Autodesk Fusion 360 part; units mm, degrees
(part 3 of 7)
  line L360 (75.0921, -60.7097) -> (75.2145, -60.5939)
  line L361 (75.2145, -60.5939) -> (75.3304, -60.4715)
  line L362 (75.3304, -60.4715) -> (75.4394, -60.343)
  line L363 (75.4394, -60.343) -> (75.6678, -60.5263)
  line L364 (75.6678, -60.5263) -> (75.7289, -60.5629)
  line L365 (75.7289, -60.5629) -> (75.7952, -60.5929)
  line L366 (75.7952, -60.5929) -> (75.865, -60.6184)
  line L367 (75.865, -60.6184) -> (75.9376, -60.6398)
  line L368 (75.9376, -60.6398) -> (76.0128, -60.6576)
  line L369 (76.0128, -60.6576) -> (76.0901, -60.672)
  line L370 (76.0901, -60.672) -> (76.1695, -60.6831)
  line L371 (76.1695, -60.6831) -> (76.2508, -60.6908)
  line L372 (76.2508, -60.6908) -> (76.3338, -60.6954)
  line L373 (76.3338, -60.6954) -> (76.4183, -60.6968)
  line L374 (76.4183, -60.6968) -> (76.5044, -60.695)
  line L375 (76.5044, -60.695) -> (76.5918, -60.69)
  line L376 (76.5918, -60.69) -> (76.66, -60.5798)
  line L377 (76.66, -60.5798) -> (76.7248, -60.4675)
  line L378 (76.7248, -60.4675) -> (76.7861, -60.3533)
  line L379 (76.7861, -60.3533) -> (76.7467, -60.2752)
  line L380 (76.7467, -60.2752) -> (76.7053, -60.1998)
  line L381 (76.7053, -60.1998) -> (76.6618, -60.1272)
  line L382 (76.6618, -60.1272) -> (76.6164, -60.0576)
  line L383 (76.6164, -60.0576) -> (76.569, -59.9911)
  line L384 (76.569, -59.9911) -> (76.5197, -59.9279)
  line L385 (76.5197, -59.9279) -> (76.4686, -59.8681)
  line L386 (76.4686, -59.8681) -> (76.4156, -59.8119)
  line L387 (76.4156, -59.8119) -> (76.3607, -59.7598)
  line L388 (76.3607, -59.7598) -> (76.3038, -59.7121)
  line L389 (76.3038, -59.7121) -> (76.2446, -59.6697)
  line L390 (76.2446, -59.6697) -> (76.1824, -59.635)
  line L391 (76.1824, -59.635) -> (75.9094, -59.5289)
  line L392 (75.9094, -59.5289) -> (75.9662, -59.3702)
  line L393 (75.9662, -59.3702) -> (76.0142, -59.2086)
  line L394 (76.0142, -59.2086) -> (76.0534, -59.0447)
  line L395 (76.0534, -59.0447) -> (76.0836, -58.8789)
  circle A0 centre (73.0295, -58.4089) radius 2.2
extrude "Extrude2" add sketch "Sketch2" along normal blind 2 separate body makes body 3 in component "CT idler 1"
combine "Combine1" operation add target body 2 tool bodies 3 makes body 4 at (74.9068, -57.2617, 40.3333) in component "CT idler 1"
ref_plane "WorkPlane1" through (0, 0, 39) normal (0, 0, 1) x (1, 0, 0) in component "CT idler 2"
sketch "Sketch1 (3)" plane through (0, 0, 39) normal (0, 0, 1) x (1, 0, 0) in component "CT idler 2"
  line L0 (68.9174, -62.2872) -> (69.364, -62.3098)
  line L1 (69.364, -62.3098) -> (69.4361, -62.3072)
  line L2 (69.4361, -62.3072) -> (69.5085, -62.2993)
  line L3 (69.5085, -62.2993) -> (69.581, -62.2878)
  line L4 (69.581, -62.2878) -> (69.6537, -62.2735)
  line L5 (69.6537, -62.2735) -> (69.7264, -62.2566)
  line L6 (69.7264, -62.2566) -> (69.7991, -62.2373)
  line L7 (69.7991, -62.2373) -> (69.8719, -62.2159)
  line L8 (69.8719, -62.2159) -> (69.9447, -62.1924)
  line L9 (69.9447, -62.1924) -> (70.0175, -62.167)
  line L10 (70.0175, -62.167) -> (70.0902, -62.1397)
  line L11 (70.0902, -62.1397) -> (70.1629, -62.1105)
  line L12 (70.1629, -62.1105) -> (70.2355, -62.0796)
  line L13 (70.2355, -62.0796) -> (70.2374, -61.9478)
  line L14 (70.2374, -61.9478) -> (70.2374, -61.816)
  line L15 (70.2374, -61.816) -> (70.2355, -61.6842)
  line L16 (70.2355, -61.6842) -> (70.1629, -61.6533)
  line L17 (70.1629, -61.6533) -> (70.0902, -61.6242)
  line L18 (70.0902, -61.6242) -> (70.0175, -61.5969)
  line L19 (70.0175, -61.5969) -> (69.9447, -61.5714)
  line L20 (69.9447, -61.5714) -> (69.8719, -61.548)
  line L21 (69.8719, -61.548) -> (69.7991, -61.5265)
  line L22 (69.7991, -61.5265) -> (69.7264, -61.5073)
  line L23 (69.7264, -61.5073) -> (69.6537, -61.4904)
  line L24 (69.6537, -61.4904) -> (69.581, -61.476)
  line L25 (69.581, -61.476) -> (69.5085, -61.4646)
  line L26 (69.5085, -61.4646) -> (69.4361, -61.4567)
  line L27 (69.4361, -61.4567) -> (69.364, -61.4541)
  line L28 (69.364, -61.4541) -> (68.9174, -61.4767)
  line L29 (68.9174, -61.4767) -> (68.9035, -61.2604)
  line L30 (68.9035, -61.2604) -> (68.8837, -61.0447)
  line L31 (68.8837, -61.0447) -> (68.8582, -60.8295)
  line L32 (68.8582, -60.8295) -> (68.8268, -60.6151)
  line L33 (68.8268, -60.6151) -> (69.2684, -60.5443)
  line L34 (69.2684, -60.5443) -> (69.3384, -60.5268)
  line L35 (69.3384, -60.5268) -> (69.4076, -60.504)
  line L36 (69.4076, -60.504) -> (69.4761, -60.4777)
  line L37 (69.4761, -60.4777) -> (69.5442, -60.4486)
  line L38 (69.5442, -60.4486) -> (69.6118, -60.4169)
  line L39 (69.6118, -60.4169) -> (69.6789, -60.383)
  line L40 (69.6789, -60.383) -> (69.7457, -60.3469)
  line L41 (69.7457, -60.3469) -> (69.812, -60.3088)
  line L42 (69.812, -60.3088) -> (69.8779, -60.2688)
  line L43 (69.8779, -60.2688) -> (69.9433, -60.2269)
  line L44 (69.9433, -60.2269) -> (70.0084, -60.1833)
  line L45 (70.0084, -60.1833) -> (70.073, -60.138)
  line L46 (70.073, -60.138) -> (70.0474, -60.0087)
  line L47 (70.0474, -60.0087) -> (70.02, -59.8798)
  line L48 (70.02, -59.8798) -> (69.9908, -59.7513)
  line L49 (69.9908, -59.7513) -> (69.9133, -59.7361)
  line L50 (69.9133, -59.7361) -> (69.8362, -59.7228)
  line L51 (69.8362, -59.7228) -> (69.7594, -59.7112)
  line L52 (69.7594, -59.7112) -> (69.6829, -59.7014)
  line L53 (69.6829, -59.7014) -> (69.6068, -59.6936)
  line L54 (69.6068, -59.6936) -> (69.5312, -59.6877)
  line L55 (69.5312, -59.6877) -> (69.456, -59.684)
  line L56 (69.456, -59.684) -> (69.3814, -59.6826)
  line L57 (69.3814, -59.6826) -> (69.3073, -59.6837)
  line L58 (69.3073, -59.6837) -> (69.234, -59.6876)
  line L59 (69.234, -59.6876) -> (69.1616, -59.6949)
  line L60 (69.1616, -59.6949) -> (69.0905, -59.7073)
  line L61 (69.0905, -59.7073) -> (68.6583, -59.8223)
  line L62 (68.6583, -59.8223) -> (68.5998, -59.6137)
  line L63 (68.5998, -59.6137) -> (68.5356, -59.4067)
  line L64 (68.5356, -59.4067) -> (68.4658, -59.2015)
  line L65 (68.4658, -59.2015) -> (68.3906, -58.9984)
  line L66 (68.3906, -58.9984) -> (68.8078, -58.8373)
  line L67 (68.8078, -58.8373) -> (68.8726, -58.8056)
  line L68 (68.8726, -58.8056) -> (68.9355, -58.7689)
  line L69 (68.9355, -58.7689) -> (68.9971, -58.729)
  line L70 (68.9971, -58.729) -> (69.0577, -58.6864)
  line L71 (69.0577, -58.6864) -> (69.1172, -58.6413)
  line L72 (69.1172, -58.6413) -> (69.1758, -58.5942)
  line L73 (69.1758, -58.5942) -> (69.2336, -58.545)
  line L74 (69.2336, -58.545) -> (69.2906, -58.4939)
  line L75 (69.2906, -58.4939) -> (69.3467, -58.4411)
  line L76 (69.3467, -58.4411) -> (69.402, -58.3865)
  line L77 (69.402, -58.3865) -> (69.4566, -58.3304)
  line L78 (69.4566, -58.3304) -> (69.5104, -58.2726)
  line L79 (69.5104, -58.2726) -> (69.4585, -58.1514)
  line L80 (69.4585, -58.1514) -> (69.4049, -58.031)
  line L81 (69.4049, -58.031) -> (69.3495, -57.9114)
  line L82 (69.3495, -57.9114) -> (69.2706, -57.9127)
  line L83 (69.2706, -57.9127) -> (69.1924, -57.9157)
  line L84 (69.1924, -57.9157) -> (69.1148, -57.9203)
  line L85 (69.1148, -57.9203) -> (69.038, -57.9266)
  line L86 (69.038, -57.9266) -> (68.9619, -57.9348)
  line L87 (68.9619, -57.9348) -> (68.8867, -57.9448)
  line L88 (68.8867, -57.9448) -> (68.8124, -57.9568)
  line L89 (68.8124, -57.9568) -> (68.7391, -57.971)
  line L90 (68.7391, -57.971) -> (68.667, -57.9874)
  line L91 (68.667, -57.9874) -> (68.5961, -58.0065)
  line L92 (68.5961, -58.0065) -> (68.5267, -58.0287)
  line L93 (68.5267, -58.0287) -> (68.4598, -58.0556)
  line L94 (68.4598, -58.0556) -> (68.0609, -58.2579)
  line L95 (68.0609, -58.2579) -> (67.9603, -58.066)
  line L96 (67.9603, -58.066) -> (67.8545, -57.8769)
  line L97 (67.8545, -57.8769) -> (67.7436, -57.6908)
  line L98 (67.7436, -57.6908) -> (67.6277, -57.5076)
  line L99 (67.6277, -57.5076) -> (68.0024, -57.2634)
  line L100 (68.0024, -57.2634) -> (68.0592, -57.2189)
  line L101 (68.0592, -57.2189) -> (68.1131, -57.17)
  line L102 (68.1131, -57.17) -> (68.1651, -57.1181)
  line L103 (68.1651, -57.1181) -> (68.2154, -57.0638)
  line L104 (68.2154, -57.0638) -> (68.2643, -57.0074)
  line L105 (68.2643, -57.0074) -> (68.3118, -56.949)
  line L106 (68.3118, -56.949) -> (68.3581, -56.8889)
  line L107 (68.3581, -56.8889) -> (68.4032, -56.8271)
  line L108 (68.4032, -56.8271) -> (68.4471, -56.7638)
  line L109 (68.4471, -56.7638) -> (68.4899, -56.6989)
  line L110 (68.4899, -56.6989) -> (68.5316, -56.6326)
  line L111 (68.5316, -56.6326) -> (68.5722, -56.5649)
  line L112 (68.5722, -56.5649) -> (68.4962, -56.4572)
  line L113 (68.4962, -56.4572) -> (68.4187, -56.3506)
  line L114 (68.4187, -56.3506) -> (68.3398, -56.2451)
  line L115 (68.3398, -56.2451) -> (68.2629, -56.2628)
  line L116 (68.2629, -56.2628) -> (68.1869, -56.2819)
  line L117 (68.1869, -56.2819) -> (68.112, -56.3026)
  line L118 (68.112, -56.3026) -> (68.0382, -56.3248)
  line L119 (68.0382, -56.3248) -> (67.9655, -56.3485)
  line L120 (67.9655, -56.3485) -> (67.894, -56.374)
  line L121 (67.894, -56.374) -> (67.8238, -56.4012)
  line L122 (67.8238, -56.4012) -> (67.7551, -56.4302)
  line L123 (67.7551, -56.4302) -> (67.6879, -56.4613)
  line L124 (67.6879, -56.4613) -> (67.6225, -56.4947)
  line L125 (67.6225, -56.4947) -> (67.5593, -56.5308)
  line L126 (67.5593, -56.5308) -> (67.4994, -56.5711)
  line L127 (67.4994, -56.5711) -> (67.1514, -56.8519)
  line L128 (67.1514, -56.8519) -> (67.013, -56.6852)
  line L129 (67.013, -56.6852) -> (66.8702, -56.5222)
  line L130 (66.8702, -56.5222) -> (66.7231, -56.3631)
  line L131 (66.7231, -56.3631) -> (66.5717, -56.2081)
  line L132 (66.5717, -56.2081) -> (66.8873, -55.8913)
  line L133 (66.8873, -55.8913) -> (66.9336, -55.836)
  line L134 (66.9336, -55.836) -> (66.9762, -55.7769)
  line L135 (66.9762, -55.7769) -> (67.0162, -55.7153)
  line L136 (67.0162, -55.7153) -> (67.0542, -55.6518)
  line L137 (67.0542, -55.6518) -> (67.0902, -55.5864)
  line L138 (67.0902, -55.5864) -> (67.1246, -55.5195)
  line L139 (67.1246, -55.5195) -> (67.1574, -55.4511)
  line L140 (67.1574, -55.4511) -> (67.1886, -55.3813)
  line L141 (67.1886, -55.3813) -> (67.2184, -55.3102)
  line L142 (67.2184, -55.3102) -> (67.2468, -55.2378)
  line L143 (67.2468, -55.2378) -> (67.2738, -55.1643)
  line L144 (67.2738, -55.1643) -> (67.2994, -55.0897)
  line L145 (67.2994, -55.0897) -> (67.2027, -55.0001)
  line L146 (67.2027, -55.0001) -> (67.1048, -54.9119)
  line L147 (67.1048, -54.9119) -> (67.0056, -54.8251)
  line L148 (67.0056, -54.8251) -> (66.934, -54.8584)
  line L149 (66.934, -54.8584) -> (66.8638, -54.8929)
  line L150 (66.8638, -54.8929) -> (66.7948, -54.9287)
  line L151 (66.7948, -54.9287) -> (66.7272, -54.9658)
  line L152 (66.7272, -54.9658) -> (66.661, -55.0041)
  line L153 (66.661, -55.0041) -> (66.5964, -55.0439)
  line L154 (66.5964, -55.0439) -> (66.5334, -55.0851)
  line L155 (66.5334, -55.0851) -> (66.4722, -55.1278)
  line L156 (66.4722, -55.1278) -> (66.4129, -55.1722)
  line L157 (66.4129, -55.1722) -> (66.3559, -55.2184)
  line L158 (66.3559, -55.2184) -> (66.3016, -55.2669)
  line L159 (66.3016, -55.2669) -> (66.2514, -55.3187)
  line L160 (66.2514, -55.3187) -> (65.9693, -55.6658)
  line L161 (65.9693, -55.6658) -> (65.7993, -55.5314)
  line L162 (65.7993, -55.5314) -> (65.6258, -55.4017)
  line L163 (65.6258, -55.4017) -> (65.4488, -55.2767)
  line L164 (65.4488, -55.2767) -> (65.2684, -55.1566)
  line L165 (65.2684, -55.1566) -> (65.5114, -54.7811)
  line L166 (65.5114, -54.7811) -> (65.5452, -54.7173)
  line L167 (65.5452, -54.7173) -> (65.5745, -54.6507)
  line L168 (65.5745, -54.6507) -> (65.6008, -54.5821)
  line L169 (65.6008, -54.5821) -> (65.6247, -54.5121)
  line L170 (65.6247, -54.5121) -> (65.6465, -54.4406)
  line L171 (65.6465, -54.4406) -> (65.6662, -54.368)
  line L172 (65.6662, -54.368) -> (65.684, -54.2943)
  line L173 (65.684, -54.2943) -> (65.7, -54.2195)
  line L174 (65.7, -54.2195) -> (65.7144, -54.1438)
  line L175 (65.7144, -54.1438) -> (65.7271, -54.0671)
  line L176 (65.7271, -54.0671) -> (65.7382, -53.9896)
  line L177 (65.7382, -53.9896) -> (65.7478, -53.9112)
  line L178 (65.7478, -53.9112) -> (65.6346, -53.8437)
  line L179 (65.6346, -53.8437) -> (65.5204, -53.7778)
  line L180 (65.5204, -53.7778) -> (65.4054, -53.7135)
  line L181 (65.4054, -53.7135) -> (65.3423, -53.761)
  line L182 (65.3423, -53.761) -> (65.2807, -53.8094)
  line L183 (65.2807, -53.8094) -> (65.2207, -53.8587)
  line L184 (65.2207, -53.8587) -> (65.1623, -53.909)
  line L185 (65.1623, -53.909) -> (65.1055, -53.9603)
  line L186 (65.1055, -53.9603) -> (65.0506, -54.0126)
  line L187 (65.0506, -54.0126) -> (64.9976, -54.066)
  line L188 (64.9976, -54.066) -> (64.9466, -54.1205)
  line L189 (64.9466, -54.1205) -> (64.8978, -54.1762)
  line L190 (64.8978, -54.1762) -> (64.8517, -54.2333)
  line L191 (64.8517, -54.2333) -> (64.8086, -54.2921)
  line L192 (64.8086, -54.2921) -> (64.7703, -54.3532)
  line L193 (64.7703, -54.3532) -> (64.5665, -54.7513)
  line L194 (64.5665, -54.7513) -> (64.3723, -54.6552)
  line L195 (64.3723, -54.6552) -> (64.1756, -54.5644)
  line L196 (64.1756, -54.5644) -> (63.9765, -54.479)
  line L197 (63.9765, -54.479) -> (63.7751, -54.399)
  line L198 (63.7751, -54.399) -> (63.9346, -53.9811)
  line L199 (63.9346, -53.9811) -> (63.9544, -53.9117)
  line L200 (63.9544, -53.9117) -> (63.9693, -53.8405)
  line L201 (63.9693, -53.8405) -> (63.9808, -53.768)
  line L202 (63.9808, -53.768) -> (63.9896, -53.6944)
  line L203 (63.9896, -53.6944) -> (63.996, -53.6201)
  line L204 (63.996, -53.6201) -> (64.0002, -53.5449)
  line L205 (64.0002, -53.5449) -> (64.0023, -53.4691)
  line L206 (64.0023, -53.4691) -> (64.0024, -53.3926)
  line L207 (64.0024, -53.3926) -> (64.0007, -53.3155)
  line L208 (64.0007, -53.3155) -> (63.9972, -53.2379)
  line L209 (63.9972, -53.2379) -> (63.992, -53.1598)
  line L210 (63.992, -53.1598) -> (63.985, -53.0812)
  line L211 (63.985, -53.0812) -> (63.8603, -53.0387)
  line L212 (63.8603, -53.0387) -> (63.7349, -52.9979)
  line L213 (63.7349, -52.9979) -> (63.609, -52.959)
  line L214 (63.609, -52.959) -> (63.5572, -53.0185)
  line L215 (63.5572, -53.0185) -> (63.507, -53.0786)
  line L216 (63.507, -53.0786) -> (63.4585, -53.1394)
  line L217 (63.4585, -53.1394) -> (63.4119, -53.2007)
  line L218 (63.4119, -53.2007) -> (63.367, -53.2627)
  line L219 (63.367, -53.2627) -> (63.3242, -53.3253)
  line L220 (63.3242, -53.3253) -> (63.2834, -53.3885)
  line L221 (63.2834, -53.3885) -> (63.2448, -53.4525)
  line L222 (63.2448, -53.4525) -> (63.2087, -53.5171)
  line L223 (63.2087, -53.5171) -> (63.1755, -53.5825)
  line L224 (63.1755, -53.5825) -> (63.1456, -53.6489)
  line L225 (63.1456, -53.6489) -> (63.1208, -53.7167)
  line L226 (63.1208, -53.7167) -> (63.0043, -54.1485)
  line L227 (63.0043, -54.1485) -> (62.7943, -54.0949)
  line L228 (62.7943, -54.0949) -> (62.583, -54.047)
  line L229 (62.583, -54.047) -> (62.3705, -54.0048)
  line L230 (62.3705, -54.0048) -> (62.1568, -53.9684)
  line L231 (62.1568, -53.9684) -> (62.226, -53.5265)
  line L232 (62.226, -53.5265) -> (62.231, -53.4545)
  line L233 (62.231, -53.4545) -> (62.2307, -53.3817)
  line L234 (62.2307, -53.3817) -> (62.2269, -53.3084)
  line L235 (62.2269, -53.3084) -> (62.2202, -53.2347)
  line L236 (62.2202, -53.2347) -> (62.211, -53.1606)
  line L237 (62.211, -53.1606) -> (62.1994, -53.0862)
  line L238 (62.1994, -53.0862) -> (62.1857, -53.0116)
  line L239 (62.1857, -53.0116) -> (62.17, -52.9368)
  line L240 (62.17, -52.9368) -> (62.1523, -52.8617)
  line L241 (62.1523, -52.8617) -> (62.1327, -52.7865)
  line L242 (62.1327, -52.7865) -> (62.1114, -52.7112)
  line L243 (62.1114, -52.7112) -> (62.0882, -52.6357)
  line L244 (62.0882, -52.6357) -> (61.9573, -52.6201)
  line L245 (61.9573, -52.6201) -> (61.8263, -52.6063)
  line L246 (61.8263, -52.6063) -> (61.695, -52.5944)
  line L247 (61.695, -52.5944) -> (61.6567, -52.6634)
  line L248 (61.6567, -52.6634) -> (61.6201, -52.7327)
  line L249 (61.6201, -52.7327) -> (61.5853, -52.8021)
  line L250 (61.5853, -52.8021) -> (61.5524, -52.8719)
  line L251 (61.5524, -52.8719) -> (61.5215, -52.9418)
  line L252 (61.5215, -52.9418) -> (61.4925, -53.0119)
  line L253 (61.4925, -53.0119) -> (61.4658, -53.0823)
  line L254 (61.4658, -53.0823) -> (61.4414, -53.1528)
  line L255 (61.4414, -53.1528) -> (61.4195, -53.2235)
  line L256 (61.4195, -53.2235) -> (61.4006, -53.2945)
  line L257 (61.4006, -53.2945) -> (61.3851, -53.3656)
  line L258 (61.3851, -53.3656) -> (61.375, -53.4371)
  line L259 (61.375, -53.4371) -> (61.3508, -53.8837)
  line L260 (61.3508, -53.8837) -> (61.1343, -53.8749)
  line L261 (61.1343, -53.8749) -> (60.9176, -53.8719)
  line L262 (60.9176, -53.8719) -> (60.701, -53.8749)
  line L263 (60.701, -53.8749) -> (60.4844, -53.8837)
  line L264 (60.4844, -53.8837) -> (60.4603, -53.4371)
  line L265 (60.4603, -53.4371) -> (60.4501, -53.3656)
  line L266 (60.4501, -53.3656) -> (60.4347, -53.2945)
  line L267 (60.4347, -53.2945) -> (60.4157, -53.2235)
  line L268 (60.4157, -53.2235) -> (60.3939, -53.1528)
  line L269 (60.3939, -53.1528) -> (60.3694, -53.0823)
  line L270 (60.3694, -53.0823) -> (60.3427, -53.0119)
  line L271 (60.3427, -53.0119) -> (60.3138, -52.9418)
  line L272 (60.3138, -52.9418) -> (60.2828, -52.8719)
  line L273 (60.2828, -52.8719) -> (60.2499, -52.8021)
  line L274 (60.2499, -52.8021) -> (60.2151, -52.7327)
  line L275 (60.2151, -52.7327) -> (60.1786, -52.6634)
  line L276 (60.1786, -52.6634) -> (60.1402, -52.5944)
  line L277 (60.1402, -52.5944) -> (60.009, -52.6063)
  line L278 (60.009, -52.6063) -> (59.8779, -52.6201)
  line L279 (59.8779, -52.6201) -> (59.747, -52.6357)
  line L280 (59.747, -52.6357) -> (59.7239, -52.7112)
  line L281 (59.7239, -52.7112) -> (59.7025, -52.7865)
  line L282 (59.7025, -52.7865) -> (59.6829, -52.8617)
  line L283 (59.6829, -52.8617) -> (59.6653, -52.9368)
  line L284 (59.6653, -52.9368) -> (59.6495, -53.0116)
  line L285 (59.6495, -53.0116) -> (59.6358, -53.0862)
  line L286 (59.6358, -53.0862) -> (59.6243, -53.1606)
  line L287 (59.6243, -53.1606) -> (59.6151, -53.2347)
  line L288 (59.6151, -53.2347) -> (59.6084, -53.3084)
  line L289 (59.6084, -53.3084) -> (59.6046, -53.3817)
  line L290 (59.6046, -53.3817) -> (59.6043, -53.4545)
  line L291 (59.6043, -53.4545) -> (59.6092, -53.5265)
  line L292 (59.6092, -53.5265) -> (59.6784, -53.9684)
  line L293 (59.6784, -53.9684) -> (59.4648, -54.0048)
  line L294 (59.4648, -54.0048) -> (59.2523, -54.047)
  line L295 (59.2523, -54.047) -> (59.0409, -54.0949)
  line L296 (59.0409, -54.0949) -> (58.831, -54.1485)
  line L297 (58.831, -54.1485) -> (58.7145, -53.7167)
  line L298 (58.7145, -53.7167) -> (58.6897, -53.6489)
  line L299 (58.6897, -53.6489) -> (58.6598, -53.5825)
  line L300 (58.6598, -53.5825) -> (58.6265, -53.5171)
  line L301 (58.6265, -53.5171) -> (58.5904, -53.4525)
  line L302 (58.5904, -53.4525) -> (58.5519, -53.3885)
  line L303 (58.5519, -53.3885) -> (58.5111, -53.3253)
  line L304 (58.5111, -53.3253) -> (58.4682, -53.2627)
  line L305 (58.4682, -53.2627) -> (58.4234, -53.2007)
  line L306 (58.4234, -53.2007) -> (58.3767, -53.1394)
  line L307 (58.3767, -53.1394) -> (58.3282, -53.0786)
  line L308 (58.3282, -53.0786) -> (58.2781, -53.0185)
  line L309 (58.2781, -53.0185) -> (58.2262, -52.959)
  line L310 (58.2262, -52.959) -> (58.1003, -52.9979)
  line L311 (58.1003, -52.9979) -> (57.975, -53.0387)
  line L312 (57.975, -53.0387) -> (57.8502, -53.0812)
  line L313 (57.8502, -53.0812) -> (57.8433, -53.1598)
  line L314 (57.8433, -53.1598) -> (57.838, -53.2379)
  line L315 (57.838, -53.2379) -> (57.8345, -53.3155)
  line L316 (57.8345, -53.3155) -> (57.8328, -53.3926)
  line L317 (57.8328, -53.3926) -> (57.833, -53.4691)
  line L318 (57.833, -53.4691) -> (57.8351, -53.5449)
  line L319 (57.8351, -53.5449) -> (57.8393, -53.6201)
  line L320 (57.8393, -53.6201) -> (57.8456, -53.6944)
  line L321 (57.8456, -53.6944) -> (57.8545, -53.768)
  line L322 (57.8545, -53.768) -> (57.866, -53.8405)
  line L323 (57.866, -53.8405) -> (57.8808, -53.9117)
  line L324 (57.8808, -53.9117) -> (57.9006, -53.9811)
  line L325 (57.9006, -53.9811) -> (58.0602, -54.399)
  line L326 (58.0602, -54.399) -> (57.8588, -54.479)
  line L327 (57.8588, -54.479) -> (57.6597, -54.5644)
  line L328 (57.6597, -54.5644) -> (57.4629, -54.6552)
  line L329 (57.4629, -54.6552) -> (57.2687, -54.7513)
  line L330 (57.2687, -54.7513) -> (57.065, -54.3532)
  line L331 (57.065, -54.3532) -> (57.0266, -54.2921)
  line L332 (57.0266, -54.2921) -> (56.9836, -54.2333)
  line L333 (56.9836, -54.2333) -> (56.9374, -54.1762)
  line L334 (56.9374, -54.1762) -> (56.8887, -54.1205)
  line L335 (56.8887, -54.1205) -> (56.8377, -54.066)
  line L336 (56.8377, -54.066) -> (56.7846, -54.0126)
  line L337 (56.7846, -54.0126) -> (56.7297, -53.9603)
  line L338 (56.7297, -53.9603) -> (56.673, -53.909)
  line L339 (56.673, -53.909) -> (56.6146, -53.8587)
  line L340 (56.6146, -53.8587) -> (56.5545, -53.8094)
  line L341 (56.5545, -53.8094) -> (56.4929, -53.761)
  line L342 (56.4929, -53.761) -> (56.4299, -53.7135)
  line L343 (56.4299, -53.7135) -> (56.3148, -53.7778)
  line L344 (56.3148, -53.7778) -> (56.2007, -53.8437)
  line L345 (56.2007, -53.8437) -> (56.0875, -53.9112)
  line L346 (56.0875, -53.9112) -> (56.097, -53.9896)
  line L347 (56.097, -53.9896) -> (56.1081, -54.0671)
  line L348 (56.1081, -54.0671) -> (56.1208, -54.1438)
  line L349 (56.1208, -54.1438) -> (56.1352, -54.2195)
  line L350 (56.1352, -54.2195) -> (56.1513, -54.2943)
  line L351 (56.1513, -54.2943) -> (56.1691, -54.368)
  line L352 (56.1691, -54.368) -> (56.1888, -54.4406)
  line L353 (56.1888, -54.4406) -> (56.2105, -54.5121)
  line L354 (56.2105, -54.5121) -> (56.2344, -54.5821)
  line L355 (56.2344, -54.5821) -> (56.2608, -54.6507)
  line L356 (56.2608, -54.6507) -> (56.2901, -54.7173)
  line L357 (56.2901, -54.7173) -> (56.3239, -54.7811)
  line L358 (56.3239, -54.7811) -> (56.5668, -55.1566)
  line L359 (56.5668, -55.1566) -> (56.3865, -55.2767)
  line L360 (56.3865, -55.2767) -> (56.2095, -55.4017)
  line L361 (56.2095, -55.4017) -> (56.0359, -55.5314)
  line L362 (56.0359, -55.5314) -> (55.8659, -55.6658)
  line L363 (55.8659, -55.6658) -> (55.5838, -55.3187)
  line L364 (55.5838, -55.3187) -> (55.5336, -55.2669)
  line L365 (55.5336, -55.2669) -> (55.4793, -55.2184)
  line L366 (55.4793, -55.2184) -> (55.4223, -55.1722)
  line L367 (55.4223, -55.1722) -> (55.363, -55.1278)
  line L368 (55.363, -55.1278) -> (55.3018, -55.0851)
  line L369 (55.3018, -55.0851) -> (55.2388, -55.0439)
  line L370 (55.2388, -55.0439) -> (55.1742, -55.0041)
  line L371 (55.1742, -55.0041) -> (55.1081, -54.9658)
  line L372 (55.1081, -54.9658) -> (55.0405, -54.9287)
  line L373 (55.0405, -54.9287) -> (54.9715, -54.8929)
  line L374 (54.9715, -54.8929) -> (54.9012, -54.8584)
  line L375 (54.9012, -54.8584) -> (54.8296, -54.8251)
  line L376 (54.8296, -54.8251) -> (54.7305, -54.9119)
  line L377 (54.7305, -54.9119) -> (54.6325, -55.0001)
  line L378 (54.6325, -55.0001) -> (54.5358, -55.0897)
  line L379 (54.5358, -55.0897) -> (54.5615, -55.1643)
  line L380 (54.5615, -55.1643) -> (54.5884, -55.2378)
  line L381 (54.5884, -55.2378) -> (54.6168, -55.3102)
  line L382 (54.6168, -55.3102) -> (54.6466, -55.3813)
  line L383 (54.6466, -55.3813) -> (54.6778, -55.4511)
  line L384 (54.6778, -55.4511) -> (54.7106, -55.5195)
  line L385 (54.7106, -55.5195) -> (54.745, -55.5864)
  line L386 (54.745, -55.5864) -> (54.7811, -55.6518)
  line L387 (54.7811, -55.6518) -> (54.819, -55.7153)
  line L388 (54.819, -55.7153) -> (54.8591, -55.7769)
  line L389 (54.8591, -55.7769) -> (54.9016, -55.836)
  line L390 (54.9016, -55.836) -> (54.9479, -55.8913)
  line L391 (54.9479, -55.8913) -> (55.2636, -56.2081)
  line L392 (55.2636, -56.2081) -> (55.1122, -56.3631)
  line L393 (55.1122, -56.3631) -> (54.965, -56.5222)
  line L394 (54.965, -56.5222) -> (54.8222, -56.6852)
  line L395 (54.8222, -56.6852) -> (54.6839, -56.8519)
  line L396 (54.6839, -56.8519) -> (54.3358, -56.5711)
  line L397 (54.3358, -56.5711) -> (54.2759, -56.5308)
  line L398 (54.2759, -56.5308) -> (54.2127, -56.4947)
  line L399 (54.2127, -56.4947) -> (54.1473, -56.4613)
  line L400 (54.1473, -56.4613) -> (54.0802, -56.4302)
  line L401 (54.0802, -56.4302) -> (54.0114, -56.4012)
  line L402 (54.0114, -56.4012) -> (53.9412, -56.374)
  line L403 (53.9412, -56.374) -> (53.8698, -56.3485)
  line L404 (53.8698, -56.3485) -> (53.7971, -56.3248)
  line L405 (53.7971, -56.3248) -> (53.7232, -56.3026)
  line L406 (53.7232, -56.3026) -> (53.6483, -56.2819)
  line L407 (53.6483, -56.2819) -> (53.5724, -56.2628)
  line L408 (53.5724, -56.2628) -> (53.4955, -56.2451)
  line L409 (53.4955, -56.2451) -> (53.4165, -56.3506)
  line L410 (53.4165, -56.3506) -> (53.339, -56.4572)
  line L411 (53.339, -56.4572) -> (53.2631, -56.5649)
  line L412 (53.2631, -56.5649) -> (53.3037, -56.6326)
  line L413 (53.3037, -56.6326) -> (53.3454, -56.6989)
  line L414 (53.3454, -56.6989) -> (53.3882, -56.7638)
  line L415 (53.3882, -56.7638) -> (53.4321, -56.8271)
  line L416 (53.4321, -56.8271) -> (53.4772, -56.8889)
  line L417 (53.4772, -56.8889) -> (53.5234, -56.949)
  line L418 (53.5234, -56.949) -> (53.571, -57.0074)
  line L419 (53.571, -57.0074) -> (53.6199, -57.0638)
  line L420 (53.6199, -57.0638) -> (53.6702, -57.1181)
  line L421 (53.6702, -57.1181) -> (53.7221, -57.17)
  line L422 (53.7221, -57.17) -> (53.776, -57.2189)
  line L423 (53.776, -57.2189) -> (53.8328, -57.2634)
  line L424 (53.8328, -57.2634) -> (54.2075, -57.5076)
  line L425 (54.2075, -57.5076) -> (54.0916, -57.6908)
  line L426 (54.0916, -57.6908) -> (53.9808, -57.8769)
  line L427 (53.9808, -57.8769) -> (53.875, -58.066)
  line L428 (53.875, -58.066) -> (53.7743, -58.2579)
  line L429 (53.7743, -58.2579) -> (53.3755, -58.0556)
  line L430 (53.3755, -58.0556) -> (53.3085, -58.0287)
  line L431 (53.3085, -58.0287) -> (53.2392, -58.0065)
  line L432 (53.2392, -58.0065) -> (53.1683, -57.9874)
  line L433 (53.1683, -57.9874) -> (53.0961, -57.971)
  line L434 (53.0961, -57.971) -> (53.0228, -57.9568)
  line L435 (53.0228, -57.9568) -> (52.9485, -57.9448)
  line L436 (52.9485, -57.9448) -> (52.8733, -57.9348)
  line L437 (52.8733, -57.9348) -> (52.7973, -57.9266)
  line L438 (52.7973, -57.9266) -> (52.7204, -57.9203)
  line L439 (52.7204, -57.9203) -> (52.6429, -57.9157)
  line L440 (52.6429, -57.9157) -> (52.5646, -57.9127)
  line L441 (52.5646, -57.9127) -> (52.4857, -57.9114)
  line L442 (52.4857, -57.9114) -> (52.4304, -58.031)
  line L443 (52.4304, -58.031) -> (52.3768, -58.1514)
  line L444 (52.3768, -58.1514) -> (52.3249, -58.2726)
  line L445 (52.3249, -58.2726) -> (52.3787, -58.3304)
  line L446 (52.3787, -58.3304) -> (52.4332, -58.3865)
  line L447 (52.4332, -58.3865) -> (52.4886, -58.4411)
  line L448 (52.4886, -58.4411) -> (52.5447, -58.4939)
  line L449 (52.5447, -58.4939) -> (52.6016, -58.545)
  line L450 (52.6016, -58.545) -> (52.6594, -58.5942)
  line L451 (52.6594, -58.5942) -> (52.718, -58.6413)
  line L452 (52.718, -58.6413) -> (52.7776, -58.6864)
  line L453 (52.7776, -58.6864) -> (52.8381, -58.729)
  line L454 (52.8381, -58.729) -> (52.8997, -58.7689)
  line L455 (52.8997, -58.7689) -> (52.9626, -58.8056)
  line L456 (52.9626, -58.8056) -> (53.0274, -58.8373)
  line L457 (53.0274, -58.8373) -> (53.4447, -58.9984)
  line L458 (53.4447, -58.9984) -> (53.3694, -59.2015)
  line L459 (53.3694, -59.2015) -> (53.2997, -59.4067)
  line L460 (53.2997, -59.4067) -> (53.2355, -59.6137)
  line L461 (53.2355, -59.6137) -> (53.1769, -59.8223)
  line L462 (53.1769, -59.8223) -> (52.7448, -59.7073)
  line L463 (52.7448, -59.7073) -> (52.6737, -59.6949)
  line L464 (52.6737, -59.6949) -> (52.6012, -59.6876)
  line L465 (52.6012, -59.6876) -> (52.5279, -59.6837)
  line L466 (52.5279, -59.6837) -> (52.4539, -59.6826)
  line L467 (52.4539, -59.6826) -> (52.3793, -59.684)
  line L468 (52.3793, -59.684) -> (52.3041, -59.6877)
  line L469 (52.3041, -59.6877) -> (52.2284, -59.6936)
  line L470 (52.2284, -59.6936) -> (52.1524, -59.7014)
  line L471 (52.1524, -59.7014) -> (52.0759, -59.7112)
  line L472 (52.0759, -59.7112) -> (51.9991, -59.7228)
  line L473 (51.9991, -59.7228) -> (51.9219, -59.7361)
  line L474 (51.9219, -59.7361) -> (51.8444, -59.7513)
  line L475 (51.8444, -59.7513) -> (51.8152, -59.8798)
  line L476 (51.8152, -59.8798) -> (51.7878, -60.0087)
  line L477 (51.7878, -60.0087) -> (51.7622, -60.138)
  line L478 (51.7622, -60.138) -> (51.8269, -60.1833)
  line L479 (51.8269, -60.1833) -> (51.8919, -60.2269)
  line L480 (51.8919, -60.2269) -> (51.9574, -60.2688)
  line L481 (51.9574, -60.2688) -> (52.0233, -60.3088)
  line L482 (52.0233, -60.3088) -> (52.0896, -60.3469)
  line L483 (52.0896, -60.3469) -> (52.1563, -60.383)
  line L484 (52.1563, -60.383) -> (52.2235, -60.4169)
  line L485 (52.2235, -60.4169) -> (52.2911, -60.4486)
  line L486 (52.2911, -60.4486) -> (52.3591, -60.4777)
  line L487 (52.3591, -60.4777) -> (52.4277, -60.504)
  line L488 (52.4277, -60.504) -> (52.4968, -60.5268)
  line L489 (52.4968, -60.5268) -> (52.5668, -60.5443)
  line L490 (52.5668, -60.5443) -> (53.0084, -60.6151)
  line L491 (53.0084, -60.6151) -> (52.9771, -60.8295)
  line L492 (52.9771, -60.8295) -> (52.9515, -61.0447)
  line L493 (52.9515, -61.0447) -> (52.9318, -61.2604)
  line L494 (52.9318, -61.2604) -> (52.9179, -61.4767)
  line L495 (52.9179, -61.4767) -> (52.4712, -61.4541)
  line L496 (52.4712, -61.4541) -> (52.3991, -61.4567)
  line L497 (52.3991, -61.4567) -> (52.3267, -61.4646)
  line L498 (52.3267, -61.4646) -> (52.2542, -61.476)
  line L499 (52.2542, -61.476) -> (52.1816, -61.4904)
  line L500 (52.1816, -61.4904) -> (52.1089, -61.5073)
  line L501 (52.1089, -61.5073) -> (52.0361, -61.5265)
  line L502 (52.0361, -61.5265) -> (51.9633, -61.548)
  line L503 (51.9633, -61.548) -> (51.8906, -61.5714)
  line L504 (51.8906, -61.5714) -> (51.8178, -61.5969)
  line L505 (51.8178, -61.5969) -> (51.745, -61.6242)
  line L506 (51.745, -61.6242) -> (51.6723, -61.6533)
  line L507 (51.6723, -61.6533) -> (51.5997, -61.6842)
  line L508 (51.5997, -61.6842) -> (51.5979, -61.816)
  line L509 (51.5979, -61.816) -> (51.5979, -61.9478)
  line L510 (51.5979, -61.9478) -> (51.5997, -62.0796)
  line L511 (51.5997, -62.0796) -> (51.6723, -62.1105)
  line L512 (51.6723, -62.1105) -> (51.745, -62.1397)
  line L513 (51.745, -62.1397) -> (51.8178, -62.167)
  line L514 (51.8178, -62.167) -> (51.8906, -62.1924)
  line L515 (51.8906, -62.1924) -> (51.9633, -62.2159)
  line L516 (51.9633, -62.2159) -> (52.0361, -62.2373)
  line L517 (52.0361, -62.2373) -> (52.1089, -62.2566)
  line L518 (52.1089, -62.2566) -> (52.1816, -62.2735)
  line L519 (52.1816, -62.2735) -> (52.2542, -62.2878)
  line L520 (52.2542, -62.2878) -> (52.3267, -62.2993)
  line L521 (52.3267, -62.2993) -> (52.3991, -62.3072)
  line L522 (52.3991, -62.3072) -> (52.4712, -62.3098)
  line L523 (52.4712, -62.3098) -> (52.9179, -62.2872)
  line L524 (52.9179, -62.2872) -> (52.9318, -62.5034)
  line L525 (52.9318, -62.5034) -> (52.9515, -62.7192)
  line L526 (52.9515, -62.7192) -> (52.9771, -62.9344)
  line L527 (52.9771, -62.9344) -> (53.0084, -63.1488)
  line L528 (53.0084, -63.1488) -> (52.5668, -63.2195)
  line L529 (52.5668, -63.2195) -> (52.4968, -63.2371)
  line L530 (52.4968, -63.2371) -> (52.4277, -63.2599)
  line L531 (52.4277, -63.2599) -> (52.3591, -63.2861)
  line L532 (52.3591, -63.2861) -> (52.2911, -63.3153)
  line L533 (52.2911, -63.3153) -> (52.2235, -63.3469)
  line L534 (52.2235, -63.3469) -> (52.1563, -63.3809)
  line L535 (52.1563, -63.3809) -> (52.0896, -63.417)
  line L536 (52.0896, -63.417) -> (52.0233, -63.4551)
  line L537 (52.0233, -63.4551) -> (51.9574, -63.4951)
  line L538 (51.9574, -63.4951) -> (51.8919, -63.5369)
  line L539 (51.8919, -63.5369) -> (51.8269, -63.5805)
  line L540 (51.8269, -63.5805) -> (51.7622, -63.6259)
  line L541 (51.7622, -63.6259) -> (51.7878, -63.7552)
  line L542 (51.7878, -63.7552) -> (51.8152, -63.8841)
  line L543 (51.8152, -63.8841) -> (51.8444, -64.0126)
  line L544 (51.8444, -64.0126) -> (51.9219, -64.0277)
  line L545 (51.9219, -64.0277) -> (51.9991, -64.0411)
  line L546 (51.9991, -64.0411) -> (52.0759, -64.0527)
  line L547 (52.0759, -64.0527) -> (52.1524, -64.0625)
  line L548 (52.1524, -64.0625) -> (52.2284, -64.0703)
  line L549 (52.2284, -64.0703) -> (52.3041, -64.0761)
  line L550 (52.3041, -64.0761) -> (52.3793, -64.0798)
  line L551 (52.3793, -64.0798) -> (52.4539, -64.0813)
  line L552 (52.4539, -64.0813) -> (52.5279, -64.0802)
  line L553 (52.5279, -64.0802) -> (52.6012, -64.0763)
  line L554 (52.6012, -64.0763) -> (52.6737, -64.069)
  line L555 (52.6737, -64.069) -> (52.7448, -64.0566)
  line L556 (52.7448, -64.0566) -> (53.1769, -63.9416)
  line L557 (53.1769, -63.9416) -> (53.2355, -64.1502)
  line L558 (53.2355, -64.1502) -> (53.2997, -64.3572)
  line L559 (53.2997, -64.3572) -> (53.3694, -64.5623)
  line L560 (53.3694, -64.5623) -> (53.4447, -64.7655)
  line L561 (53.4447, -64.7655) -> (53.0274, -64.9265)
  line L562 (53.0274, -64.9265) -> (52.9626, -64.9583)
  line L563 (52.9626, -64.9583) -> (52.8997, -64.9949)
  line L564 (52.8997, -64.9949) -> (52.8381, -65.0349)
  line L565 (52.8381, -65.0349) -> (52.7776, -65.0775)
  line L566 (52.7776, -65.0775) -> (52.718, -65.1225)
  line L567 (52.718, -65.1225) -> (52.6594, -65.1697)
  line L568 (52.6594, -65.1697) -> (52.6016, -65.2189)
  line L569 (52.6016, -65.2189) -> (52.5447, -65.2699)
  line L570 (52.5447, -65.2699) -> (52.4886, -65.3228)
  line L571 (52.4886, -65.3228) -> (52.4332, -65.3773)
  line L572 (52.4332, -65.3773) -> (52.3787, -65.4335)
  line L573 (52.3787, -65.4335) -> (52.3249, -65.4913)
  line L574 (52.3249, -65.4913) -> (52.3768, -65.6124)
  line L575 (52.3768, -65.6124) -> (52.4304, -65.7328)
  line L576 (52.4304, -65.7328) -> (52.4857, -65.8525)
  line L577 (52.4857, -65.8525) -> (52.5646, -65.8511)
  line L578 (52.5646, -65.8511) -> (52.6429, -65.8482)
  line L579 (52.6429, -65.8482) -> (52.7204, -65.8436)
  line L580 (52.7204, -65.8436) -> (52.7973, -65.8372)
  line L581 (52.7973, -65.8372) -> (52.8733, -65.8291)
  line L582 (52.8733, -65.8291) -> (52.9485, -65.819)
  line L583 (52.9485, -65.819) -> (53.0228, -65.807)
  line L584 (53.0228, -65.807) -> (53.0961, -65.7929)
  line L585 (53.0961, -65.7929) -> (53.1683, -65.7765)
  line L586 (53.1683, -65.7765) -> (53.2392, -65.7574)
  line L587 (53.2392, -65.7574) -> (53.3085, -65.7352)
  line L588 (53.3085, -65.7352) -> (53.3755, -65.7083)
  line L589 (53.3755, -65.7083) -> (53.7743, -65.5059)
  line L590 (53.7743, -65.5059) -> (53.875, -65.6978)
  line L591 (53.875, -65.6978) -> (53.9808, -65.8869)
  line L592 (53.9808, -65.8869) -> (54.0916, -66.0731)
  line L593 (54.0916, -66.0731) -> (54.2075, -66.2562)
  line L594 (54.2075, -66.2562) -> (53.8328, -66.5004)
  line L595 (53.8328, -66.5004) -> (53.776, -66.545)
  line L596 (53.776, -66.545) -> (53.7221, -66.5939)
  line L597 (53.7221, -66.5939) -> (53.6702, -66.6458)
  line L598 (53.6702, -66.6458) -> (53.6199, -66.7001)
  line L599 (53.6199, -66.7001) -> (53.571, -66.7565)
  line L600 (53.571, -66.7565) -> (53.5234, -66.8148)
  line L601 (53.5234, -66.8148) -> (53.4772, -66.8749)
  line L602 (53.4772, -66.8749) -> (53.4321, -66.9367)
  line L603 (53.4321, -66.9367) -> (53.3882, -67.0001)
  line L604 (53.3882, -67.0001) -> (53.3454, -67.0649)
  line L605 (53.3454, -67.0649) -> (53.3037, -67.1312)
  line L606 (53.3037, -67.1312) -> (53.2631, -67.1989)
  line L607 (53.2631, -67.1989) -> (53.339, -67.3066)
  line L608 (53.339, -67.3066) -> (53.4165, -67.4133)
  line L609 (53.4165, -67.4133) -> (53.4955, -67.5188)
  line L610 (53.4955, -67.5188) -> (53.5724, -67.5011)
  line L611 (53.5724, -67.5011) -> (53.6483, -67.4819)
  line L612 (53.6483, -67.4819) -> (53.7232, -67.4613)
  line L613 (53.7232, -67.4613) -> (53.7971, -67.4391)
  line L614 (53.7971, -67.4391) -> (53.8698, -67.4153)
  line L615 (53.8698, -67.4153) -> (53.9412, -67.3899)
  line L616 (53.9412, -67.3899) -> (54.0114, -67.3627)
  line L617 (54.0114, -67.3627) -> (54.0802, -67.3336)
  line L618 (54.0802, -67.3336) -> (54.1473, -67.3025)
  line L619 (54.1473, -67.3025) -> (54.2127, -67.2692)
  line L620 (54.2127, -67.2692) -> (54.2759, -67.233)
  line L621 (54.2759, -67.233) -> (54.3358, -67.1928)
  line L622 (54.3358, -67.1928) -> (54.6839, -66.9119)
  line L623 (54.6839, -66.9119) -> (54.8222, -67.0787)
  line L624 (54.8222, -67.0787) -> (54.965, -67.2417)
  line L625 (54.965, -67.2417) -> (55.1122, -67.4007)
  line L626 (55.1122, -67.4007) -> (55.2636, -67.5557)
  line L627 (55.2636, -67.5557) -> (54.9479, -67.8725)
  line L628 (54.9479, -67.8725) -> (54.9016, -67.9279)
  line L629 (54.9016, -67.9279) -> (54.8591, -67.987)
  line L630 (54.8591, -67.987) -> (54.819, -68.0485)
  line L631 (54.819, -68.0485) -> (54.7811, -68.1121)
  line L632 (54.7811, -68.1121) -> (54.745, -68.1774)
  line L633 (54.745, -68.1774) -> (54.7106, -68.2444)
  line L634 (54.7106, -68.2444) -> (54.6778, -68.3128)
  line L635 (54.6778, -68.3128) -> (54.6466, -68.3826)
  line L636 (54.6466, -68.3826) -> (54.6168, -68.4537)
  line L637 (54.6168, -68.4537) -> (54.5884, -68.526)
  line L638 (54.5884, -68.526) -> (54.5615, -68.5996)
  line L639 (54.5615, -68.5996) -> (54.5358, -68.6742)
  line L640 (54.5358, -68.6742) -> (54.6325, -68.7638)
  line L641 (54.6325, -68.7638) -> (54.7305, -68.852)
  line L642 (54.7305, -68.852) -> (54.8296, -68.9388)
  line L643 (54.8296, -68.9388) -> (54.9012, -68.9055)
  line L644 (54.9012, -68.9055) -> (54.9715, -68.8709)
  line L645 (54.9715, -68.8709) -> (55.0405, -68.8352)
  line L646 (55.0405, -68.8352) -> (55.1081, -68.7981)
  line L647 (55.1081, -68.7981) -> (55.1742, -68.7597)
  line L648 (55.1742, -68.7597) -> (55.2388, -68.72)
  line L649 (55.2388, -68.72) -> (55.3018, -68.6788)
  line L650 (55.3018, -68.6788) -> (55.363, -68.6361)
  line L651 (55.363, -68.6361) -> (55.4223, -68.5917)
  line L652 (55.4223, -68.5917) -> (55.4793, -68.5455)
  line L653 (55.4793, -68.5455) -> (55.5336, -68.497)
  line L654 (55.5336, -68.497) -> (55.5838, -68.4451)
  line L655 (55.5838, -68.4451) -> (55.8659, -68.0981)
  line L656 (55.8659, -68.0981) -> (56.0359, -68.2324)
  line L657 (56.0359, -68.2324) -> (56.2095, -68.3622)
  line L658 (56.2095, -68.3622) -> (56.3865, -68.4871)
  line L659 (56.3865, -68.4871) -> (56.5668, -68.6073)
  line L660 (56.5668, -68.6073) -> (56.3239, -68.9828)
  line L661 (56.3239, -68.9828) -> (56.2901, -69.0466)
  line L662 (56.2901, -69.0466) -> (56.2608, -69.1132)
  line L663 (56.2608, -69.1132) -> (56.2344, -69.1817)
  line L664 (56.2344, -69.1817) -> (56.2105, -69.2518)
  line L665 (56.2105, -69.2518) -> (56.1888, -69.3232)
  line L666 (56.1888, -69.3232) -> (56.1691, -69.3958)
  line L667 (56.1691, -69.3958) -> (56.1513, -69.4696)
  line L668 (56.1513, -69.4696) -> (56.1352, -69.5444)
  line L669 (56.1352, -69.5444) -> (56.1208, -69.6201)
  line L670 (56.1208, -69.6201) -> (56.1081, -69.6968)
  line L671 (56.1081, -69.6968) -> (56.097, -69.7743)
  line L672 (56.097, -69.7743) -> (56.0875, -69.8526)
  line L673 (56.0875, -69.8526) -> (56.2007, -69.9201)
  line L674 (56.2007, -69.9201) -> (56.3148, -69.986)
  line L675 (56.3148, -69.986) -> (56.4299, -70.0503)
  line L676 (56.4299, -70.0503) -> (56.4929, -70.0029)
  line L677 (56.4929, -70.0029) -> (56.5545, -69.9545)
  line L678 (56.5545, -69.9545) -> (56.6146, -69.9051)
  line L679 (56.6146, -69.9051) -> (56.673, -69.8548)
  line L680 (56.673, -69.8548) -> (56.7297, -69.8036)
  line L681 (56.7297, -69.8036) -> (56.7846, -69.7512)
  line L682 (56.7846, -69.7512) -> (56.8377, -69.6979)
  line L683 (56.8377, -69.6979) -> (56.8887, -69.6433)
  line L684 (56.8887, -69.6433) -> (56.9374, -69.5876)
  line L685 (56.9374, -69.5876) -> (56.9836, -69.5305)
  line L686 (56.9836, -69.5305) -> (57.0266, -69.4718)
  line L687 (57.0266, -69.4718) -> (57.065, -69.4107)
  line L688 (57.065, -69.4107) -> (57.2687, -69.0125)
  line L689 (57.2687, -69.0125) -> (57.4629, -69.1086)
  line L690 (57.4629, -69.1086) -> (57.6597, -69.1994)
  line L691 (57.6597, -69.1994) -> (57.8588, -69.2849)
  line L692 (57.8588, -69.2849) -> (58.0602, -69.3649)
  line L693 (58.0602, -69.3649) -> (57.9006, -69.7827)
  line L694 (57.9006, -69.7827) -> (57.8808, -69.8521)
  line L695 (57.8808, -69.8521) -> (57.866, -69.9234)
  line L696 (57.866, -69.9234) -> (57.8545, -69.9959)
  line L697 (57.8545, -69.9959) -> (57.8456, -70.0694)
  line L698 (57.8456, -70.0694) -> (57.8393, -70.1438)
  line L699 (57.8393, -70.1438) -> (57.8351, -70.2189)
  line L700 (57.8351, -70.2189) -> (57.833, -70.2948)
  line L701 (57.833, -70.2948) -> (57.8328, -70.3712)
  line L702 (57.8328, -70.3712) -> (57.8345, -70.4483)
  line L703 (57.8345, -70.4483) -> (57.838, -70.5259)
  line L704 (57.838, -70.5259) -> (57.8433, -70.6041)
  line L705 (57.8433, -70.6041) -> (57.8502, -70.6827)
  line L706 (57.8502, -70.6827) -> (57.975, -70.7252)
  line L707 (57.975, -70.7252) -> (58.1003, -70.7659)
  line L708 (58.1003, -70.7659) -> (58.2262, -70.8049)
  line L709 (58.2262, -70.8049) -> (58.2781, -70.7453)
  line L710 (58.2781, -70.7453) -> (58.3282, -70.6852)
  line L711 (58.3282, -70.6852) -> (58.3767, -70.6245)
  line L712 (58.3767, -70.6245) -> (58.4234, -70.5631)
  line L713 (58.4234, -70.5631) -> (58.4682, -70.5012)
  line L714 (58.4682, -70.5012) -> (58.5111, -70.4386)
  line L715 (58.5111, -70.4386) -> (58.5519, -70.3753)
  line L716 (58.5519, -70.3753) -> (58.5904, -70.3114)
  line L717 (58.5904, -70.3114) -> (58.6265, -70.2468)
  line L718 (58.6265, -70.2468) -> (58.6598, -70.1813)
  line L719 (58.6598, -70.1813) -> (58.6897, -70.1149)
  line L720 (58.6897, -70.1149) -> (58.7145, -70.0472)
  line L721 (58.7145, -70.0472) -> (58.831, -69.6154)
  line L722 (58.831, -69.6154) -> (59.0409, -69.669)
  line L723 (59.0409, -69.669) -> (59.2523, -69.7169)
  line L724 (59.2523, -69.7169) -> (59.4648, -69.7591)
  line L725 (59.4648, -69.7591) -> (59.6784, -69.7955)
  line L726 (59.6784, -69.7955) -> (59.6092, -70.2373)
  line L727 (59.6092, -70.2373) -> (59.6043, -70.3093)
  line L728 (59.6043, -70.3093) -> (59.6046, -70.3821)
  line L729 (59.6046, -70.3821) -> (59.6084, -70.4555)
  line L730 (59.6084, -70.4555) -> (59.6151, -70.5292)
  line L731 (59.6151, -70.5292) -> (59.6243, -70.6033)
  line L732 (59.6243, -70.6033) -> (59.6358, -70.6776)
  line L733 (59.6358, -70.6776) -> (59.6495, -70.7523)
  line L734 (59.6495, -70.7523) -> (59.6653, -70.8271)
  line L735 (59.6653, -70.8271) -> (59.6829, -70.9021)
  line L736 (59.6829, -70.9021) -> (59.7025, -70.9773)
  line L737 (59.7025, -70.9773) -> (59.7239, -71.0527)
  line L738 (59.7239, -71.0527) -> (59.747, -71.1281)
  line L739 (59.747, -71.1281) -> (59.8779, -71.1438)
  line L740 (59.8779, -71.1438) -> (60.009, -71.1575)
  line L741 (60.009, -71.1575) -> (60.1402, -71.1695)
  line L742 (60.1402, -71.1695) -> (60.1786, -71.1005)
  line L743 (60.1786, -71.1005) -> (60.2151, -71.0312)
  line L744 (60.2151, -71.0312) -> (60.2499, -70.9617)
  line L745 (60.2499, -70.9617) -> (60.2828, -70.892)
  line L746 (60.2828, -70.892) -> (60.3138, -70.8221)
  line L747 (60.3138, -70.8221) -> (60.3427, -70.7519)
  line L748 (60.3427, -70.7519) -> (60.3694, -70.6816)
  line L749 (60.3694, -70.6816) -> (60.3939, -70.6111)
  line L750 (60.3939, -70.6111) -> (60.4157, -70.5403)
  line L751 (60.4157, -70.5403) -> (60.4347, -70.4694)
  line L752 (60.4347, -70.4694) -> (60.4501, -70.3982)
  line L753 (60.4501, -70.3982) -> (60.4603, -70.3268)
  line L754 (60.4603, -70.3268) -> (60.4844, -69.8802)
  line L755 (60.4844, -69.8802) -> (60.701, -69.889)
  line L756 (60.701, -69.889) -> (60.9176, -69.8919)
  line L757 (60.9176, -69.8919) -> (61.1343, -69.889)
  line L758 (61.1343, -69.889) -> (61.3508, -69.8802)
  line L759 (61.3508, -69.8802) -> (61.375, -70.3268)
  line L760 (61.375, -70.3268) -> (61.3851, -70.3982)
  line L761 (61.3851, -70.3982) -> (61.4006, -70.4694)
  line L762 (61.4006, -70.4694) -> (61.4195, -70.5403)
  line L763 (61.4195, -70.5403) -> (61.4414, -70.6111)
  line L764 (61.4414, -70.6111) -> (61.4658, -70.6816)
  line L765 (61.4658, -70.6816) -> (61.4925, -70.7519)
  line L766 (61.4925, -70.7519) -> (61.5215, -70.8221)
  line L767 (61.5215, -70.8221) -> (61.5524, -70.892)
  line L768 (61.5524, -70.892) -> (61.5853, -70.9617)
  line L769 (61.5853, -70.9617) -> (61.6201, -71.0312)
  line L770 (61.6201, -71.0312) -> (61.6567, -71.1005)
  line L771 (61.6567, -71.1005) -> (61.695, -71.1695)
  line L772 (61.695, -71.1695) -> (61.8263, -71.1575)
  line L773 (61.8263, -71.1575) -> (61.9573, -71.1438)
  line L774 (61.9573, -71.1438) -> (62.0882, -71.1281)
  line L775 (62.0882, -71.1281) -> (62.1114, -71.0527)
  line L776 (62.1114, -71.0527) -> (62.1327, -70.9773)
  line L777 (62.1327, -70.9773) -> (62.1523, -70.9021)
  line L778 (62.1523, -70.9021) -> (62.17, -70.8271)
  line L779 (62.17, -70.8271) -> (62.1857, -70.7523)
  line L780 (62.1857, -70.7523) -> (62.1994, -70.6776)
  line L781 (62.1994, -70.6776) -> (62.211, -70.6033)
  line L782 (62.211, -70.6033) -> (62.2202, -70.5292)
  line L783 (62.2202, -70.5292) -> (62.2269, -70.4555)
  line L784 (62.2269, -70.4555) -> (62.2307, -70.3821)
  line L785 (62.2307, -70.3821) -> (62.231, -70.3093)
  line L786 (62.231, -70.3093) -> (62.226, -70.2373)
  line L787 (62.226, -70.2373) -> (62.1568, -69.7955)
  line L788 (62.1568, -69.7955) -> (62.3705, -69.7591)
  line L789 (62.3705, -69.7591) -> (62.583, -69.7169)
  line L790 (62.583, -69.7169) -> (62.7943, -69.669)
  line L791 (62.7943, -69.669) -> (63.0043, -69.6154)
  line L792 (63.0043, -69.6154) -> (63.1208, -70.0472)
  line L793 (63.1208, -70.0472) -> (63.1456, -70.1149)
  line L794 (63.1456, -70.1149) -> (63.1755, -70.1813)
  line L795 (63.1755, -70.1813) -> (63.2087, -70.2468)
  line L796 (63.2087, -70.2468) -> (63.2448, -70.3114)
  line L797 (63.2448, -70.3114) -> (63.2834, -70.3753)
  line L798 (63.2834, -70.3753) -> (63.3242, -70.4386)
  line L799 (63.3242, -70.4386) -> (63.367, -70.5012)
  line L800 (63.367, -70.5012) -> (63.4119, -70.5631)
  line L801 (63.4119, -70.5631) -> (63.4585, -70.6245)
  line L802 (63.4585, -70.6245) -> (63.507, -70.6852)
  line L803 (63.507, -70.6852) -> (63.5572, -70.7453)
  line L804 (63.5572, -70.7453) -> (63.609, -70.8049)
  line L805 (63.609, -70.8049) -> (63.7349, -70.7659)
  line L806 (63.7349, -70.7659) -> (63.8603, -70.7252)
  line L807 (63.8603, -70.7252) -> (63.985, -70.6827)
  line L808 (63.985, -70.6827) -> (63.992, -70.6041)
  line L809 (63.992, -70.6041) -> (63.9972, -70.5259)
  line L810 (63.9972, -70.5259) -> (64.0007, -70.4483)
  line L811 (64.0007, -70.4483) -> (64.0024, -70.3712)
  line L812 (64.0024, -70.3712) -> (64.0023, -70.2948)
  line L813 (64.0023, -70.2948) -> (64.0002, -70.2189)
  line L814 (64.0002, -70.2189) -> (63.996, -70.1438)
  line L815 (63.996, -70.1438) -> (63.9896, -70.0694)
  line L816 (63.9896, -70.0694) -> (63.9808, -69.9959)
  line L817 (63.9808, -69.9959) -> (63.9693, -69.9234)
  line L818 (63.9693, -69.9234) -> (63.9544, -69.8521)
  line L819 (63.9544, -69.8521) -> (63.9346, -69.7827)
  line L820 (63.9346, -69.7827) -> (63.7751, -69.3649)
  line L821 (63.7751, -69.3649) -> (63.9765, -69.2849)
  line L822 (63.9765, -69.2849) -> (64.1756, -69.1994)
  line L823 (64.1756, -69.1994) -> (64.3723, -69.1086)
  line L824 (64.3723, -69.1086) -> (64.5665, -69.0125)
  line L825 (64.5665, -69.0125) -> (64.7703, -69.4107)
  line L826 (64.7703, -69.4107) -> (64.8086, -69.4718)
  line L827 (64.8086, -69.4718) -> (64.8517, -69.5305)
  line L828 (64.8517, -69.5305) -> (64.8978, -69.5876)
  line L829 (64.8978, -69.5876) -> (64.9466, -69.6433)
  line L830 (64.9466, -69.6433) -> (64.9976, -69.6979)
  line L831 (64.9976, -69.6979) -> (65.0506, -69.7512)
  line L832 (65.0506, -69.7512) -> (65.1055, -69.8036)
  line L833 (65.1055, -69.8036) -> (65.1623, -69.8548)
  line L834 (65.1623, -69.8548) -> (65.2207, -69.9051)
  line L835 (65.2207, -69.9051) -> (65.2807, -69.9545)
  line L836 (65.2807, -69.9545) -> (65.3423, -70.0029)
  line L837 (65.3423, -70.0029) -> (65.4054, -70.0503)
  line L838 (65.4054, -70.0503) -> (65.5204, -69.986)
  line L839 (65.5204, -69.986) -> (65.6346, -69.9201)
  line L840 (65.6346, -69.9201) -> (65.7478, -69.8526)
  line L841 (65.7478, -69.8526) -> (65.7382, -69.7743)
  line L842 (65.7382, -69.7743) -> (65.7271, -69.6968)
  line L843 (65.7271, -69.6968) -> (65.7144, -69.6201)
  line L844 (65.7144, -69.6201) -> (65.7, -69.5444)
  line L845 (65.7, -69.5444) -> (65.684, -69.4696)
  line L846 (65.684, -69.4696) -> (65.6662, -69.3958)
  line L847 (65.6662, -69.3958) -> (65.6465, -69.3232)
  line L848 (65.6465, -69.3232) -> (65.6247, -69.2518)
  line L849 (65.6247, -69.2518) -> (65.6008, -69.1817)
  line L850 (65.6008, -69.1817) -> (65.5745, -69.1132)
  line L851 (65.5745, -69.1132) -> (65.5452, -69.0466)
  line L852 (65.5452, -69.0466) -> (65.5114, -68.9828)
  line L853 (65.5114, -68.9828) -> (65.2684, -68.6073)
  line L854 (65.2684, -68.6073) -> (65.4488, -68.4871)
  line L855 (65.4488, -68.4871) -> (65.6258, -68.3622)
  line L856 (65.6258, -68.3622) -> (65.7993, -68.2324)
  line L857 (65.7993, -68.2324) -> (65.9693, -68.0981)
  line L858 (65.9693, -68.0981) -> (66.2514, -68.4451)
  line L859 (66.2514, -68.4451) -> (66.3016, -68.497)
  line L860 (66.3016, -68.497) -> (66.3559, -68.5455)
  line L861 (66.3559, -68.5455) -> (66.4129, -68.5917)
  line L862 (66.4129, -68.5917) -> (66.4722, -68.6361)
  line L863 (66.4722, -68.6361) -> (66.5334, -68.6788)
  line L864 (66.5334, -68.6788) -> (66.5964, -68.72)
  line L865 (66.5964, -68.72) -> (66.661, -68.7597)
  line L866 (66.661, -68.7597) -> (66.7272, -68.7981)
  line L867 (66.7272, -68.7981) -> (66.7948, -68.8352)
  line L868 (66.7948, -68.8352) -> (66.8638, -68.8709)
  line L869 (66.8638, -68.8709) -> (66.934, -68.9055)
  line L870 (66.934, -68.9055) -> (67.0056, -68.9388)